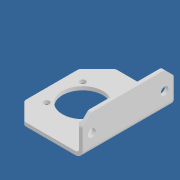
# Autodesk Inventor part: Belt_Unit_Motor_Holder
Saved by Autodesk Inventor 2020 (Build 240168000, 168)
## iProperties
Created: 2021-05-12
Part Number: Belt_Unit_Motor_Holder
Material: 一般
Document SubType Name: Sheet Metal
Designer: ken113
Density: 1 g/cm^3
Sheet Metal Rule: Default_mm
Appearance: 既定
Author: ken113
Autodesk Inventor part; units mm, degrees
ref_plane "YZ Plane" through (0, 0, 0) normal (1, 0, 0) x (0, 1, 0)
ref_plane "XZ Plane" through (0, 0, 0) normal (0, 1, 0) x (-1, 0, 0)
ref_plane "XY Plane" through (0, 0, 0) normal (0, 0, 1) x (1, 0, 0)
sketch "スケッチ1" plane through (0, 0, 0) normal (0, 1, 0) x (-1, 0, 0)
  line L0 (0, -25) -> (42, -25)
  line L1 (42, -25) -> (42, 25)
  line L2 (42, 25) -> (0, 25)
  line L3 (0, 25) -> (0, -25)
  point P0 (0, 0)
  dimension "d0" = 42
  dimension "d1" = 50
  dimension "d40" = 25
  measures "d0" distance of L1.end L2.end
  measures "d1" distance of L2.end L0.start
  measures "d40" distance from line of point (0, 0) L2
extrude "プレート1" add sketch "スケッチ1" along normal blind 2
sketch "スケッチ4" plane through (0, 2, 0) normal (0, 1, 0) x (1, 0, 0)
  circle A0 centre (-25, 0) radius 11.1
  line L0 (0, 25) -> (0, -25) projected
  point P0 (0, 0)
  dimension "d23" = 22.2
  dimension "d24" = 25
  constraints: 1 centre point
  measures "d23" diameter of A0
  measures "d24" distance from line of A0.centre L0
extrude "押し出し1" cut sketch "スケッチ4" against normal blind 10
sketch "スケッチ5" plane through (0, 2, 0) normal (0, 1, 0) x (1, 0, 0)
  circle A0 centre (-25, 0) radius 11.1 projected
  line L0 (0, 25) -> (0, -25) projected
  line L1 (-42, 25) -> (0, 25) projected
  line L2 (-42, -25) -> (-42, 25) projected
  line L3 (0, -25) -> (-42, -25) projected
  circle A1 centre (-25, 0) radius 14
  point P0 (0, 0)
  point P1 (-34.8995, -9.8995)
  point P2 (-15.1005, -9.8995)
  point P3 (-15.1005, 9.8995)
  point P4 (-34.8995, 9.8995)
  dimension "d28" = 28
  dimension "d31" = 360
  constraints: 1 coincident, 1 horizontal alignment, 8 other
hole "穴2" at (-34.8995, 2, 9.8995) at (-15.1005, 2, 9.8995) at (-15.1005, 2, -9.8995) at (-34.8995, 2, -9.8995) direction (0, -1, 0) diameter 3.2 end through all
sketch "スケッチ10" plane through (-2, 0, -25) normal (1, 0, 0) x (0, 1, 0)
  line L0 (0, 50) -> (0, 0)
  line L1 (0, 0) -> (20, 0)
  line L2 (20, 0) -> (20, 50)
  line L3 (20, 50) -> (0, 50)
  constraints: 6 end point, 1 horizontal, 1 perpendicular, 1 vertical
edge flange "フランジ4" height 20 angle 90 thickness 2 bend radius 2 thickness toward (1, 0, 0) relief tear relief width 2 relief depth 1 edges at (0, 2, 0) wall of the first edge with corners at (-2, 0, 25) (-2, 0, -25) (-2, 20, -25) (-2, 20, 25)
bend "曲げ4"
corner "コーナー4"
sketch "スケッチ12" plane through (-2, 20, -25) normal (-1, 0, 0) x (0, 0, 1)
  line L0 (0, -16) -> (50, -16) projected
  line L1 (50, -16) -> (50, 0) projected
  line L2 (50, 0) -> (0, 0) projected
  line L3 (0, -16) -> (0, 0) projected
  line L4 (45, -10) -> (5, -10)
  point P0 (25, -20)
  point P1 (25, -10)
  dimension "d77" = 40
  dimension "d78" = 10
  dimension "d79" = 25
  dimension "d80" = 50
  constraints: 2 end point, 1 horizontal, 1 horizontal alignment, 1 midpoint
  measures "d77" distance of L4.start L4.end
  measures "d78" distance from line of L2 L4.end
  measures "d79" distance from line of L3 point (25, -10)
  measures "d80" distance of L1.end L2.end
hole "穴3" at (-2, 10, -20) at (-2, 10, 20) direction (1, 0, 0) diameter 4.2 end through all
chamfer "面取り1" distance 10 angle 45 2 edges at (-42, 1, 25) (-42, 1, -25)
fillet "フィレット1" radius 2 4 edges at (-32, 1, -25) (-42, 1, -15) (-42, 1, 15) (-32, 1, 25)
chamfer "面取り2" distance 5 angle 45 2 edges at (-1, 20, -25) (-1, 20, 25)
fillet "フィレット2" radius 2 4 edges at (-1, 15, -25) (-1, 20, -20) (-1, 20, 20) (-1, 15, 25)
equation "\"d38\" = Thickness"
equation "\"d79\" = 0.5 * d80"
equation "\"d86\" = Thickness"
equation "\"d2\" = Thickness"
equation "\"d67\" = BendReliefWidth"
equation "\"d68\" = BendReliefDepth"
equation "\"d69\" = MinimumRemnant"
equation "\"d70\" = TransitionRadius"
equation "\"d73\" = BendRadius"
equation "\"d74\" = CornerReliefSize"
equation "\"d75\" = GapSize"
equation "\"d76\" = JacobiRadiusSize"
equation "\"d40\" = 0.5 * d1"
equation "\"BendRadius\" = Thickness"
equation "\"BendReliefWidth\" = Thickness"
equation "\"BendReliefDepth\" = 0.5 * Thickness"
equation "\"CornerReliefSize\" = 4 * Thickness"
equation "\"MinimumRemnant\" = 2 * Thickness"
equation "\"TransitionRadius\" = BendRadius"
equation "\"JacobiRadiusSize\" = BendRadius"
equation "\"GapSize\" = Thickness"
equation "\"Thickness\" = 2"
